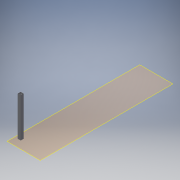
# Autodesk Inventor part: Pata
Saved by Autodesk Inventor 2016 (Build 200138000, 138)
## iProperties
Created: 2018-06-24
Part Number: Pata
Material: Generic
Document SubType Name: Modeling
Designer: damia
Density: 1 g/cm^3
Appearance: Default
Author: damia
Autodesk Inventor part; units mm, degrees
ref_plane "YZ Plane" through (0, 0, 0) normal (1, 0, 0) x (0, 1, 0)
ref_plane "XZ Plane" through (0, 0, 0) normal (0, 1, 0) x (-1, 0, 0)
ref_plane "XY Plane" through (0, 0, 0) normal (0, 0, 1) x (1, 0, 0)
ref_plane "Work Plane1" through (0, 0, 0) normal (0, 0, 1) x (1, 0, 0)
sketch "Sketch1" plane through (0, 0, 0) normal (0, 0, 1) x (1, 0, 0)
  line L0 (-250, -1000) -> (250, -1000) projected
  line L1 (250, -1000) -> (250, 1000) projected
  line L2 (250, 1000) -> (-250, 1000) projected
  line L3 (-250, 1000) -> (-250, -1000) projected
  line L4 (-223, -975) -> (-177, -975)
  line L5 (-175, -973) -> (-175, -927)
  line L6 (-177, -925) -> (-223, -925)
  line L7 (-225, -927) -> (-225, -973)
  arc A0 (-225, -973) -> (-223, -975) centre (-223, -973) ccw
  arc A1 (-223, -925) -> (-225, -927) centre (-223, -927) ccw
  arc A2 (-177, -975) -> (-175, -973) centre (-177, -973) ccw
  arc A3 (-175, -927) -> (-177, -925) centre (-177, -927) ccw
  line L8 (-223.4, -973) -> (-223.4, -927)
  arc A4 (-223, -926.6) -> (-223.4, -927) centre (-223, -927) ccw
  line L9 (-223, -926.6) -> (-177, -926.6)
  arc A5 (-176.6, -927) -> (-177, -926.6) centre (-177, -927) ccw
  line L10 (-176.6, -927) -> (-176.6, -973)
  arc A6 (-177, -973.4) -> (-176.6, -973) centre (-177, -973) ccw
  line L11 (-177, -973.4) -> (-223, -973.4)
  arc A7 (-223.4, -973) -> (-223, -973.4) centre (-223, -973) ccw
  point P0 (0, 0)
  point P1 (-175, -925)
  point P2 (-225, -925)
  dimension "d0" = 50
  dimension "d1" = 25
  dimension "d2" = 25
  dimension "d3" = 2
  dimension "d4" = 1.6
  constraints: 16 end point, 16 point on circle, 8 centre point, 8 tangent, 4 parallel, 4 point on line, 3 equal radius, 3 perpendicular, 1 horizontal, 7 other
  measures "d0" distance of point (-175, -925) point (-225, -925)
  measures "d1" distance between parallel lines of L7 L3
  measures "d2" distance between parallel lines of L0 L4
  measures "d3" radius of A0
  measures "d4" distance between parallel lines of L7 L8
extrude "Extrusion1" add sketch "Sketch1" along normal blind 650 contours A0 L7 A1 L6 A3 L5 A2 L4
body "Solid1"
